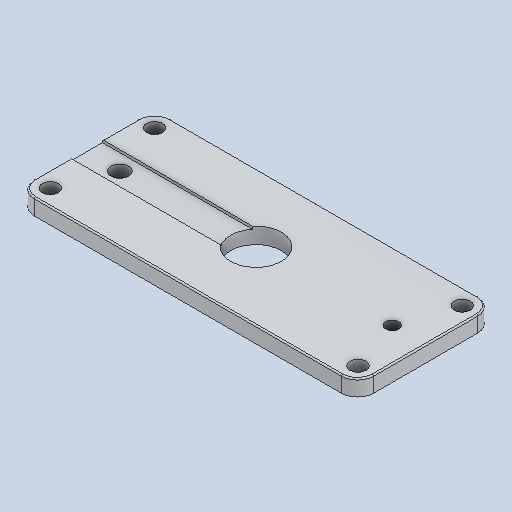
# Autodesk Inventor part: base_plate
Saved by Autodesk Inventor 2022.2 (Build 262287010, 287A)
## iProperties
Created: 2022-05-04
Part Number: base_plate
Material: Aluminum 6061-AHC
Document SubType Name: Modeling
Designer: 19710060
Density: 2.7 g/cm^3
Appearance: Aluminum - Dark
Author: 19710060
Autodesk Inventor part; units mm, degrees
ref_plane "YZ Plane" through (0, 0, 0) normal (1, 0, 0) x (0, 1, 0)
ref_plane "XZ Plane" through (0, 0, 0) normal (0, 1, 0) x (-1, 0, 0)
ref_plane "XY Plane" through (0, 0, 0) normal (0, 0, 1) x (1, 0, 0)
sketch "Esboço1" plane through (0, 0, 0) normal (0, 1, 0) x (-1, 0, 0)
  line L0 (0, 0) -> (-127, 0)
  line L1 (-127, 0) -> (-127, -51)
  line L2 (-127, -51) -> (0, -51)
  line L3 (0, -51) -> (0, 0)
  dimension "d0" = 127
  dimension "d1" = 51
  constraints: 8 end point, 2 parallel, 1 horizontal, 1 perpendicular
  measures "d0" distance of L2.end L1.end
  measures "d1" distance of L1.end L0.end
extrude "Extrusão1" add sketch "Esboço1" against normal blind 6
sketch "Esboço2" plane through (0, 0, 0) normal (0, 1, 0) x (1, 0, 0)
  line L0 (127, 51) -> (127, 0) projected
  line L1 (63.5, 0) -> (6, 0)
  line L2 (0, 51) -> (127, 51) projected
  line L3 (0, 6) -> (6, 6)
  point P0 (6, 45)
  point P1 (121.2, 45)
  point P2 (121.2, 6)
  dimension "d4" = 57.5
  constraints: 4 end point, 1 coincident
  measures "d4" distance of L1.start L1.end
hole "Furo1" at (6, 0, -6) at (6, 0, -45) at (121.2, 0, -45) at (121.2, 0, -6) direction (0, -1, 0) diameter 6 end through all
sketch "Esboço3" plane through (0, 0, 0) normal (0, 1, 0) x (1, 0, 0)
  line L0 (127, 0) -> (0, 0) projected
  line L1 (0, 0) -> (57.5, 0)
  line L2 (0, 51) -> (127, 51) projected
  line L3 (0, 0) -> (0, 51) projected
  line L4 (0, 25.5) -> (127, 25.5)
  line L5 (127, 51) -> (127, 0) projected
  line L6 (0, 25.5) -> (63.5, 25.5)
  circle A0 centre (63.5, 25.5) radius 9.5
  point P0 (57.5, 25.5)
  dimension "d17" = 57.5
  dimension "d47" = 63.5
  dimension "d48" = 19
  constraints: 6 end point, 3 midpoint, 2 point on line, 1 centre point, 1 coincident
  measures "d17" distance of L0.end L1.end
  measures "d47" distance of L4.start L6.end
  measures "d48" diameter of A0
hole "Furo2" at (63.5, 0, -25.5) direction (0, -1, 0) diameter 19 end through all
sketch "Esboço4" plane through (0, 0, 0) normal (0, 1, 0) x (1, 0, 0)
  line L0 (0, 0) -> (0, 51) projected
  line L1 (0, 31.5) -> (56.1345, 31.5)
  line L2 (0, 19.5) -> (56.1345, 19.5)
  circle A0 centre (63.5, 25.5) radius 9.5 projected
  circle A1 centre (63.5, 25.5) radius 9.5
  constraints: 4 end point, 2 point on circle, 1 centre point, 1 coincident
extrude "Extrusão2" cut sketch "Esboço4" against normal blind 1 contours L0 L1 A0 L2
sketch "Esboço5" plane through (0, -1, 0) normal (0, 1, 0) x (1, 0, 0)
  circle A0 centre (63.5, 25.5) radius 9.5 projected
  circle A1 centre (63.5, 25.5) radius 9.5
  line L0 (63.5, 25.5) -> (12.5, 25.5)
  point P0 (0, 0)
  dimension "d49" = 51
  constraints: 2 end point, 1 centre point, 1 coincident, 1 horizontal
  measures "d49" distance of L0.start L0.end
hole "Furo3" at (12.5, -1, -25.5) direction (0, -1, 0) diameter 4.917 end through all thread size "M6x1" class "6H" standard "ANSI Metric M Profile"
fillet "Arredondamento1" radius 6 4 edges at (127, -3, -51) (127, -3, 0) (0, -3, 0) (0, -3, -51)
fillet "Arredondamento2" radius 0.5 9 edges at (1.7574, 0, -49.2426) (0, 0, -38.25) (125.2426, 0, -49.2426) (127, 0, -25.5) (125.2426, 0, -1.7574) (63.5, 0, 0) (1.7574, 0, -1.7574) (0, 0, -12.75) (63.5, 0, -51)
sketch "Esboço6" plane through (0, 0, 0) normal (0, 1, 0) x (1, 0, 0)
  circle A0 centre (12.5, 25.5) radius 2.4585 projected
  circle A1 centre (12.5, 25.5) radius 2.4585
  line L0 (12.5, 25.5) -> (114.5, 25.5)
  point P0 (0, 0)
  dimension "d50" = 102
  constraints: 2 coincident, 2 end point, 1 centre point, 1 horizontal
  measures "d50" distance of L0.start L0.end
hole "Furo4" at (114.5, 0, -25.5) direction (0, -1, 0) diameter 4.917 end through all thread size "M6x1" class "6H" standard "ANSI Metric M Profile"
sketch "Sketch7" plane through (0, -6, 0) normal (0, -1, 0) x (1, 0, 0)
  point P0 (12.5, -25.5)
hole "Hole5" at (12.5, -6, -25.5) direction (0, 1, 0) diameter 6.6 end through all
